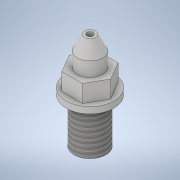
# Autodesk Inventor part: ZKE-Term-Sprung-17.5mm
Saved by Autodesk Inventor 2021 (Build 250183000, 183)
## iProperties
Created: 2020-06-09
Part Number: ZKE-Term-Sprung-17.5mm
Material: Generic
Document SubType Name: Modeling
Designer: lucas
Density: 1 g/cm^3
Appearance: Default
Project: 4Wire
Author: lucas
Revision Number: ZKE_17MM
Autodesk Inventor part; units mm, degrees
ref_plane "YZ Plane" through (0, 0, 0) normal (1, 0, 0) x (0, 1, 0)
ref_plane "XZ Plane" through (0, 0, 0) normal (0, 1, 0) x (-1, 0, 0)
sketch "Sketch1" plane through (0, 0, 0) normal (0, 1, 0) x (-1, 0, 0)
  circle A0 centre (0, 0) radius 4
  dimension "d0" = 8
  constraints: 1 centre point
  measures "d0" diameter of A0
extrude "Extrusion1" add sketch "Sketch1" along normal blind 4.5
ref_plane "Work Plane1" through (0, 9, 0) normal (0, 1, 0) x (1, 0, 0)
sketch "Sketch2" plane through (0, 9, 0) normal (0, 1, 0) x (1, 0, 0)
  circle A0 centre (0, 0) radius 1.75
  dimension "d4" = 3.5
  constraints: 1 centre point
  measures "d4" diameter of A0
loft "Loft1" add profiles "Sketch2" section 1 edges at (4, 4.5, 0)
sketch "Sketch3" plane through (0, 9, 0) normal (0, 1, 0) x (1, 0, 0)
  circle A0 centre (0, 0) radius 1
  dimension "d9" = 2
  constraints: 1 centre point
  measures "d9" diameter of A0
sketch "Sketch4" plane through (0, 0, 0) normal (0, -1, 0) x (1, 0, 0)
  circle A0 centre (0, 0) radius 1.75 projected
  line L0 (6.5, 0) -> (3.25, -5.6292)
  line L1 (3.25, -5.6292) -> (-3.25, -5.6292)
  line L2 (-3.25, -5.6292) -> (-6.5, 0)
  line L3 (-6.5, 0) -> (-3.25, 5.6292)
  line L4 (-3.25, 5.6292) -> (3.25, 5.6292)
  line L5 (3.25, 5.6292) -> (6.5, 0)
  constraints: 12 end point, 1 coincident, 13 other
extrude "Extrusion2" add sketch "Sketch4" along normal blind 5.5
sketch "Sketch5" plane through (0, -5.5, 0) normal (0, -1, 0) x (1, 0, 0)
  circle A0 centre (0, 0) radius 7.5
  dimension "d12" = 15
  constraints: 1 centre point
  measures "d12" diameter of A0
extrude "Extrusion3" add sketch "Sketch5" along normal blind 2
sketch "Sketch6" plane through (0, -7.5, 0) normal (0, -1, 0) x (1, 0, 0)
  circle A0 centre (0, 0) radius 5
  dimension "d15" = 10
  constraints: 1 centre point
  measures "d15" diameter of A0
extrude "Extrusion4" add sketch "Sketch6" along normal blind 14
thread "Thread1" size "M10x1.5" class "6g" standard "ANSI Metric M Profile" full length
extrude "Extrusion5" cut sketch "Sketch3" against normal up to surface (30.5 mm away)
body "Solid1"
